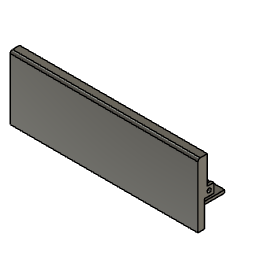
앞 범퍼 (Autodesk Fusion 360 design; units mm, degrees)
Autodesk Fusion 360 part; units mm, degrees
note: some values were not read from the file. Set by a fixed rule: which sketch regions a step uses.
sketch "스케치1" plane through (0, 0, 0) normal (1, 0, 0) x (0, 1, 0)
  line L0 (0, 0) -> (-7, 0)
  line L1 (-7, 0) -> (-7, 68)
  line L2 (-7, 68) -> (0, 68)
  line L3 (0, 68) -> (0, 0)
  line L4 (0, 0) -> (-4, 0)
  line L5 (-4, 0) -> (-4, 68)
  line L6 (-4, 68) -> (0, 68)
  line L7 (0, 68) -> (0, 0)
  dimension "d1" = 7
  dimension "d2" = 68
  dimension "d3" = 4
  constraint horizontal L0
  constraint vertical L1
  constraint horizontal L2
  constraint vertical L3
  constraint coincident L0.start L3.end
  constraint horizontal L4
  constraint vertical L5
  constraint horizontal L6
  constraint vertical L7
  measures "d1" distance of L0.start L0.end
  measures "d2" distance of L0.start L2.end
  measures "d3" distance of L0.start L4.end
extrude "돌출1" add sketch "스케치1" along normal blind 200
sketch "스케치2" plane through (0, 0, 0) normal (0, 1, 0) x (-1, 0, 0)
  line L0 (0, 0) -> (0, 68)
  line L1 (0, 68) -> (-200, 68)
  line L2 (-200, 68) -> (-200, 0)
  line L3 (-200, 0) -> (0, 0)
  line L4 (-200, 68) -> (-197, 68)
  line L5 (-197, 68) -> (-197, 65)
  line L6 (-197, 65) -> (-200, 65)
  line L7 (-200, 65) -> (-200, 68)
  line L8 (0, 0) -> (-3, 0)
  line L9 (-3, 0) -> (-3, 3)
  line L10 (-3, 3) -> (0, 3)
  line L11 (0, 3) -> (0, 0)
  line L12 (-3, 3) -> (-197, 3)
  line L13 (-197, 3) -> (-197, 65)
  line L14 (-197, 65) -> (-3, 65)
  line L15 (-3, 65) -> (-3, 3)
  dimension "d6" = 3
  dimension "d7" = 3
  dimension "d8" = 3
  constraint horizontal L4
  constraint vertical L5
  constraint horizontal L6
  constraint vertical L7
  constraint coincident L1.end L2.start
  constraint horizontal L8
  constraint vertical L9
  constraint horizontal L10
  constraint vertical L11
  constraint coincident L0.start L3.end
  constraint horizontal L12
  constraint vertical L13
  constraint horizontal L14
  constraint vertical L15
  measures "d6" distance of L1.end L4.end
  measures "d7" distance of L1.end L6.end
  measures "d8" distance of L0.start L8.end
extrude "돌출2" cut sketch "스케치2" against normal blind 4 contours L12 L13 L14 L15
sketch "스케치3" plane through (0, 0, 0) normal (0, 1, 0) x (-1, 0, 0)
  line L0 (-197, 3) -> (-197, 65)
  line L1 (-197, 65) -> (-3, 65)
  line L2 (-3, 65) -> (-3, 3)
  line L3 (-3, 3) -> (-197, 3)
  line L4 (0, 0) -> (0, 68)
  line L5 (0, 68) -> (-200, 68)
  line L6 (-200, 68) -> (-200, 0)
  line L7 (-200, 0) -> (0, 0)
  line L8 (-197, 3) -> (-177.5, 3)
  line L9 (-177.5, 3) -> (-157.5, 3)
  line L10 (-157.5, 3) -> (-157.5, 0)
  line L11 (-157.5, 0) -> (-177.5, 0)
  line L12 (-177.5, 0) -> (-177.5, 3)
  line L13 (-3, 3) -> (-22.5, 3)
  line L14 (-22.5, 3) -> (-42.5, 3)
  line L15 (-42.5, 3) -> (-42.5, 0)
  line L16 (-42.5, 0) -> (-22.5, 0)
  line L17 (-22.5, 0) -> (-22.5, 3)
  dimension "d11" = 19.5
  dimension "d12" = 20
  dimension "d13" = 19.5
  dimension "d14" = 20
  dimension "d15" = 3
  constraint coincident L0.start L3.end
  constraint perpendicular L0 L8
  constraint horizontal L9
  constraint vertical L10
  constraint horizontal L11
  constraint vertical L12
  constraint coincident L2.end L3.start
  constraint perpendicular L2 L13
  constraint horizontal L14
  constraint vertical L15
  constraint horizontal L16
  constraint vertical L17
  measures "d11" distance of L0.start L8.end
  measures "d12" distance of L8.end L9.end
  measures "d13" distance of L2.end L13.end
  measures "d14" distance of L13.end L14.end
  measures "d15" distance of L13.end L16.end
extrude "돌출3" add sketch "스케치3" along normal blind 44 contours L3 L7 L9 L10 L11 L12 | L3 L7 L14 L15 L16 L17
sketch "스케치4" plane through (0, 0, 3) normal (0, 0, 1) x (-1, 0, 0)
  line L0 (-22.5, 0) -> (-3, 0)
  line L1 (-3, 0) -> (-3, 4)
  line L2 (-3, 4) -> (-197, 4)
  line L3 (-197, 4) -> (-197, 0)
  line L4 (-197, 0) -> (-177.5, 0)
  line L5 (-177.5, 0) -> (-177.5, -44)
  line L6 (-177.5, -44) -> (-157.5, -44)
  line L7 (-157.5, -44) -> (-157.5, 0)
  line L8 (-157.5, 0) -> (-42.5, 0)
  line L9 (-42.5, 0) -> (-42.5, -44)
  line L10 (-42.5, -44) -> (-22.5, -44)
  line L11 (-22.5, -44) -> (-22.5, 0)
  line L12 (-177.5, -44) -> (-167.5, -44)
  line L13 (-167.5, -44) -> (-167.5, -34)
  line L14 (-167.5, -34) -> (-177.5, -34)
  line L15 (-177.5, -34) -> (-177.5, -44)
  line L16 (-42.5, -44) -> (-32.5, -44)
  line L17 (-32.5, -44) -> (-32.5, -34)
  line L18 (-32.5, -34) -> (-42.5, -34)
  line L19 (-42.5, -34) -> (-42.5, -44)
  circle A0 centre (-167.5, -34) radius 2.65
  circle A1 centre (-32.5, -34) radius 2.65
  dimension "d18" = 10
  dimension "d19" = 10
  dimension "d20" = 10
  dimension "d21" = 10
  dimension "d22" = 5.3
  dimension "d23" = 5.3
  constraint horizontal L12
  constraint vertical L13
  constraint horizontal L14
  constraint vertical L15
  constraint coincident L5.end L6.start
  constraint horizontal L16
  constraint vertical L17
  constraint horizontal L18
  constraint vertical L19
  constraint coincident L9.end L10.start
  constraint coincident L13.end L14.start
  constraint coincident L17.end L18.start
  measures "d18" distance of L5.end L12.end
  measures "d19" distance of L5.end L14.end
  measures "d20" distance of L9.end L16.end
  measures "d21" distance of L9.end L18.end
  measures "d22" diameter of A0
  measures "d23" diameter of A1
extrude "돌출4" cut sketch "스케치4" against normal blind 3 contours L17 L18 A1 | L17 L18 A1 | L13 L14 A0 | L13 L14 A0
fillet "필렛1" radius 2.5 1 edges at (100, -7, 68)
sketch "스케치5" plane through (0, 0, 0) normal (0, 1, 0) x (-1, 0, 0)
  line L0 (-177.5, 0) -> (-177.5, 3)
  line L1 (-177.5, 3) -> (-197, 3)
  line L2 (-197, 3) -> (-197, 65)
  line L3 (-197, 65) -> (-3, 65)
  line L4 (-3, 65) -> (-3, 3)
  line L5 (-3, 3) -> (-22.5, 3)
  line L6 (-22.5, 3) -> (-22.5, 0)
  line L7 (-22.5, 0) -> (0, 0)
  line L8 (0, 0) -> (0, 68)
  line L9 (0, 68) -> (-200, 68)
  line L10 (-200, 68) -> (-200, 0)
  line L11 (-200, 0) -> (-177.5, 0)
  line L12 (-197, 3) -> (-200, 3)
  line L13 (-200, 3) -> (-200, 38)
  line L14 (-200, 38) -> (-197, 38)
  line L15 (-197, 38) -> (-197, 3)
  line L16 (-200, 38) -> (-197, 38)
  line L17 (-197, 38) -> (-197, 28)
  line L18 (-197, 28) -> (-200, 28)
  line L19 (-200, 28) -> (-200, 38)
  line L20 (-3, 3) -> (0, 3)
  line L21 (0, 3) -> (0, 38)
  line L22 (0, 38) -> (-3, 38)
  line L23 (-3, 38) -> (-3, 3)
  line L24 (0, 38) -> (-3, 38)
  line L25 (-3, 38) -> (-3, 28)
  line L26 (-3, 28) -> (0, 28)
  line L27 (0, 28) -> (0, 38)
  dimension "d28" = 3
  dimension "d29" = 35
  dimension "d30" = 10
  dimension "d31" = 35
  dimension "d32" = 10
  constraint horizontal L12
  constraint vertical L13
  constraint horizontal L14
  constraint vertical L15
  constraint coincident L1.end L2.start
  constraint horizontal L16
  constraint vertical L17
  constraint horizontal L18
  constraint vertical L19
  constraint horizontal L20
  constraint vertical L21
  constraint horizontal L22
  constraint vertical L23
  constraint coincident L4.end L5.start
  constraint horizontal L24
  constraint vertical L25
  constraint horizontal L26
  constraint vertical L27
  measures "d28" distance of L1.end L12.end
  measures "d29" distance of L1.end L14.end
  measures "d30" distance of L13.end L18.end
  measures "d31" distance of L4.end L22.end
  measures "d32" distance of L21.end L26.end
extrude "돌출5" add sketch "스케치5" along normal blind 10 contours L2 L10 L13 L14 L15 L16 L17 L18 L19 | L4 L8 L21 L22 L23 L24 L25 L26 L27
sketch "스케치6" plane through (200, 0, 0) normal (1, 0, 0) x (0, 1, 0)
  arc A0 (-4.5, 68) -> (-7, 65.5) centre (-4.5, 65.5) ccw
  line L0 (-7, 65.5) -> (-7, 0)
  line L1 (-7, 0) -> (0, 0)
  line L2 (0, 0) -> (0, 28)
  line L3 (0, 28) -> (10, 28)
  line L4 (10, 28) -> (10, 38)
  line L5 (10, 38) -> (0, 38)
  line L6 (0, 38) -> (0, 68)
  line L7 (0, 68) -> (-4.5, 68)
  line L8 (10, 38) -> (5, 38)
  line L9 (5, 38) -> (5, 33)
  line L10 (5, 33) -> (10, 33)
  line L11 (10, 33) -> (10, 38)
  circle A1 centre (5, 33) radius 2.15
  dimension "d35" = 5
  dimension "d36" = 5
  dimension "d37" = 4.3
  constraint horizontal L8
  constraint vertical L9
  constraint horizontal L10
  constraint vertical L11
  constraint coincident L4.end L5.start
  constraint coincident L9.end L10.start
  measures "d35" distance of L4.end L8.end
  measures "d36" distance of L4.end L10.end
  measures "d37" diameter of A1
extrude "돌출6" cut sketch "스케치6" against normal blind 260 contours L9 L10 A1 | L9 L10 A1
extrude "돌출7" add 1 faces at (67.6667, 0, 67) along direction (0, 1, 0) blind 3
